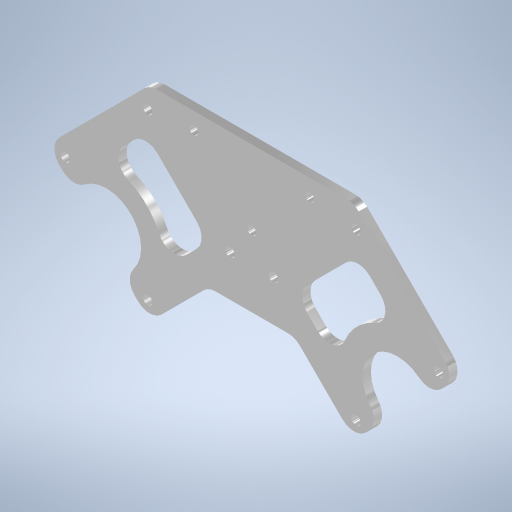
# Autodesk Inventor part: hipjoint
Saved by Autodesk Inventor 2024.1 (Build 281209000, 209)
## iProperties
Created: 2024-02-12
Part Number: hipjoint
Material: アルミニウム 6061
Document SubType Name: Modeling
Designer: hibik
Density: 2.7 g/cm^3
Appearance: アルミニウム - フラット
Author: hibik
Autodesk Inventor part; units mm, degrees
ref_plane "YZ Plane" through (0, 0, 0) normal (1, 0, 0) x (0, 1, 0)
ref_plane "XZ Plane" through (0, 0, 0) normal (0, 1, 0) x (-1, 0, 0)
ref_plane "XY Plane" through (0, 0, 0) normal (0, 0, 1) x (1, 0, 0)
sketch "スケッチ1" plane through (0, 0, 0) normal (0, 0, 1) x (1, 0, 0)
  line L0 (-18.3848, 26.163) -> (18.3848, 26.163)
  line L1 (18.3848, 26.163) -> (18.3848, 0)
  line L2 (18.3848, 0) -> (-18.3848, 0)
  line L3 (-18.3848, 0) -> (-18.3848, 26.163)
  line L4 (0, -17.9605) -> (0, 33.5169) projected
  line L5 (18.3848, 26.163) -> (0, 7.7782)
  line L6 (0, 7.7782) -> (16.9706, -9.1924)
  line L7 (16.9706, -9.1924) -> (35.3553, 9.1924)
  line L8 (35.3553, 9.1924) -> (18.3848, 26.163)
  line L9 (-18.3848, 26.163) -> (0, 7.7782)
  line L10 (0, 7.7782) -> (-16.9706, -9.1924)
  line L11 (-16.9706, -9.1924) -> (-35.3553, 9.1924)
  line L12 (-35.3553, 9.1924) -> (-18.3848, 26.163)
  circle A0 centre (-26.163, 0) radius 6.25
  circle A1 centre (26.163, 0) radius 6.25
  line L13 (-35.3553, 9.1924) -> (-16.9706, -9.1924)
  line L14 (-16.9706, -9.1924) -> (-18.3848, -10.6066)
  line L15 (-18.3848, -10.6066) -> (-36.7696, 7.7782)
  line L16 (-36.7696, 7.7782) -> (-35.3553, 9.1924)
  line L17 (35.3553, 9.1924) -> (16.9706, -9.1924)
  line L18 (16.9706, -9.1924) -> (18.3848, -10.6066)
  line L19 (18.3848, -10.6066) -> (36.7696, 7.7782)
  line L20 (36.7696, 7.7782) -> (35.3553, 9.1924)
  line L21 (-51.4774, 0) -> (51.4774, 0) projected
  circle A2 centre (26.163, 0) radius 10.25
  circle A3 centre (-26.163, 0) radius 10.25
  line L22 (31.8198, 5.6569) -> (20.5061, -5.6569)
  line L23 (20.5061, -5.6569) -> (7.7782, 7.0711)
  line L24 (7.7782, 7.0711) -> (19.0919, 18.3848)
  line L25 (19.0919, 18.3848) -> (31.8198, 5.6569)
  line L26 (-31.8198, 5.6569) -> (-20.5061, -5.6569)
  line L27 (-20.5061, -5.6569) -> (-7.7782, 7.0711)
  line L28 (-7.7782, 7.0711) -> (-19.0919, 18.3848)
  line L29 (-19.0919, 18.3848) -> (-31.8198, 5.6569)
  point P0 (0, 0)
  point P1 (0, 26.163)
  point P2 (-31.7642, 2.7728)
  point P3 (-23.3901, -5.6012)
  point P4 (-7.7782, 0)
  point P5 (7.7782, 0)
  point P6 (23.3901, -5.6012)
  point P7 (31.7642, 2.7728)
  point P8 (14.8492, 0)
  point P9 (27.2887, 10.188)
  point P10 (15.913, 0)
  point P11 (-15.913, 0)
  point P12 (-27.2887, 10.188)
  point P13 (-14.8492, 0)
  dimension "d0" = 26
  dimension "d1" = 24
  dimension "d2" = 12.5
  dimension "d3" = 12.5
  dimension "d4" = 2
  dimension "d5" = 2
  dimension "d6" = 45
  dimension "d7" = 45
  dimension "d14" = 4
  dimension "d15" = 4
  dimension "d16" = 5
  dimension "d17" = 5
  dimension "d18" = 6
  dimension "d19" = 5
  dimension "d20" = 5
  dimension "d21" = 6
  constraints: 56 end point, 16 equal length, 8 perpendicular, 7 point on line, 5 midpoint, 4 centre point, 1 coincident, 1 collinear, 1 horizontal
  measures "d0" distance between parallel lines of L10 L12
  measures "d1" distance between parallel lines of L9 L11
  measures "d2" diameter of A0
  measures "d3" diameter of A1
  measures "d4" distance between parallel lines of L15 L13
  measures "d5" distance between parallel lines of L19 L7
  measures "d6" angle of L0 L12
  measures "d7" angle of L0 L8
  measures "d14" radial gap between concentric circles of A2 A1
  measures "d15" radial gap between concentric circles of A3 A0
  measures "d16" distance between parallel lines of L8 L25
  measures "d17" distance between parallel lines of L6 L23
  measures "d18" distance between parallel lines of L5 L24
  measures "d19" distance between parallel lines of L12 L29
  measures "d20" distance between parallel lines of L10 L27
  measures "d21" distance between parallel lines of L9 L28
extrude "押し出し1" add sketch "スケッチ1" along normal blind 1.5 contours L9 L10 L2 L27 L28 L3 | L0 L4 L9 | L3 L28 L29 A3 L11 L12 | L0 L5 L4 | L6 L2 L4 | L5 L1 L24 L23 L2 L6 | L4 L2 L10 | L11 A3 L15 L16 | L8 L7 A2 L25 L24 L1 | A3 L2 L3 | L3 L21 A0 L11 L29 A3 | L2 L23 A2 L7 L6 | L10 L11 A3 L27 L2 | A3 L29 L11 | L11 A0 L15 A3 | L20 L19 A2 L7 | L2 A3 L27 L11 A0 L21 | L2 L27 A3 | L2 A2 L23 | L7 A2 L19 L18 | L14 L15 A3 L11 | A2 L25 L7 A1 L21 L1 | L1 L2 A2 | A2 L19 A1 L7 | L7 L25 A2 | A3 L11 L27 | L2 L21 A1 L7 L23 A2 | L23 L7 A2 | L7 A1 L19 A2 | A3 L15 A0 L11
fillet "フィレット1" radius 3 22 edges at (-18.3848, -10.6066, 0.75) (-23.3901, -5.6012, 0.75) (-31.7642, 2.7728, 0.75) (-36.7696, 7.7782, 0.75) (-18.3848, 26.163, 0.75) (18.3848, 26.163, 0.75) (36.7696, 7.7782, 0.75) (31.7642, 2.7728, 0.75) (23.3901, -5.6012, 0.75) (18.3848, -10.6066, 0.75) (-7.7782, 0, 0.75) (7.7782, 0, 0.75) (27.2887, 10.188, 0.75) (15.913, 0, 0.75) (14.8492, 0, 0.75) (7.7782, 7.0711, 0.75) (19.0919, 18.3848, 0.75) (-7.7782, 7.0711, 0.75) (-19.0919, 18.3848, 0.75) (-27.2887, 10.188, 0.75) (-15.913, 0, 0.75) (-14.8492, 0, 0.75)
sketch "スケッチ2" plane through (0, 0, 1.5) normal (0, 0, 1) x (1, 0, 0)
  circle A0 centre (18.7383, 22.2739) radius 0.85 projected
  circle A1 centre (33.5876, 7.4246) radius 0.85 projected
  circle A2 centre (18.7383, -7.4246) radius 0.85 projected
  circle A3 centre (3.8891, 7.4246) radius 0.85 projected
  circle A4 centre (-18.7383, 22.2739) radius 0.85 projected
  circle A5 centre (-33.5876, 7.4246) radius 0.85 projected
  circle A6 centre (-18.7383, -7.4246) radius 0.85 projected
  circle A7 centre (-3.8891, 7.4246) radius 0.85 projected
  point P0 (0, 0)
extrude "押し出し2" cut sketch "スケッチ2" against normal through all
sketch "スケッチ3" plane through (0, 0, 0) normal (0, 0, -1) x (-1, 0, 0)
  point P0 (0, 0)
sketch "スケッチ4" plane through (0, 0, 0) normal (0, 0, -1) x (-1, 0, 0)
  line L0 (-17.1421, 26.163) -> (17.1421, 26.163) projected
  line L1 (-17.6777, 26.163) -> (0, 8.4853)
  line L2 (0, 8.4853) -> (17.6777, 26.163)
  line L3 (17.6777, 26.163) -> (-17.6777, 26.163)
  line L4 (-17.6777, 26.163) -> (-22.0303, 21.8103)
  line L5 (0, 8.4853) -> (-1.4365, 7.0488)
  line L6 (6.5355, 0) -> (-6.5355, 0) projected
  circle A0 centre (-10.435, 23.163) radius 0.8
  circle A1 centre (10.435, 23.163) radius 0.8
  circle A2 centre (0, 12.7279) radius 0.8
  point P0 (0, 0)
  point P1 (0, 26.163)
  point P2 (0, 0)
  dimension "d22" = 25
  dimension "d23" = 45
  dimension "d24" = 1.6
  dimension "d25" = 1.6
  dimension "d26" = 1.6
  dimension "d27" = 3
  dimension "d28" = 3
  dimension "d29" = 3
  dimension "d30" = 3
  dimension "d31" = 3
  constraints: 11 end point, 3 centre point, 3 perpendicular, 2 midpoint, 1 horizontal, 1 horizontal alignment, 1 point on line, 1 vertical alignment
  measures "d22" distance between parallel lines of L5 L4
  measures "d23" angle of L0 L1
  measures "d24" diameter of A0
  measures "d25" diameter of A1
  measures "d26" diameter of A2
  measures "d27" distance from line of L0 A0.centre
  measures "d28" distance from line of L1 A0.centre
  measures "d29" distance from line of L2 A1.centre
  measures "d30" distance from line of L2 A2.centre
  measures "d31" distance from line of L1 A2.centre
extrude "押し出し3" cut sketch "スケッチ4" against normal through all contours A0 | A1 | A2
equation "\"d5\" = d4"
equation "\"d7\" = d6"
